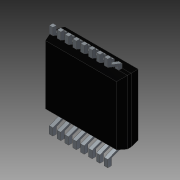
# Autodesk Inventor part: LTC6905
Saved by Autodesk Inventor 2013 (Build 170138000, 138)
## iProperties
Created: 2015-07-03
Part Number: LTC6905
Material: Ogólny
Document SubType Name: Modeling
Designer: terg
Density: 1 g/cm^3
Author: terg
Autodesk Inventor part; units mm, degrees
ref_plane "YZ Plane" through (0, 0, 0) normal (1, 0, 0) x (0, 1, 0)
ref_plane "XZ Plane" through (0, 0, 0) normal (0, 1, 0) x (-1, 0, 0)
sketch "Szkic1" plane through (0, 0, 0) normal (0, 1, 0) x (-1, 0, 0)
  line L0 (0, 0) -> (6.3, 0)
  line L1 (6.3, 0) -> (6.3, 5.3)
  line L2 (6.3, 5.3) -> (0, 5.3)
  line L3 (0, 5.3) -> (0, 0)
  dimension "d0" = 6.3
  dimension "d1" = 5.3
  constraints: 8 end point, 2 parallel, 1 horizontal, 1 perpendicular
  measures "d0" distance of L2.end L1.end
  measures "d1" distance of L1.end L0.end
extrude "Wyciągnięcie proste1" add sketch "Szkic1" along normal blind 1.7
chamfer "Faza1" distance 0.1 distance2 0.7 1 edges at (-3.15, 1.7, 0) measured on face at (-3.15, 1.7, 0.5)
chamfer "Faza2" distance 0.1 distance2 0.7 1 edges at (-3.15, 1.7, 5.3) measured on face at (-3.15, 1.7, 4.8)
chamfer "Faza3" distance 0.1 distance2 0.7 1 edges at (-6.3, 1.7, 2.65) measured on face at (-5.8, 1.7, 2.65)
chamfer "Faza4" distance 0.1 distance2 0.7 1 edges at (0, 1.7, 2.65) measured on face at (-0.5, 1.7, 2.65)
chamfer "Faza5" distance 0.7 distance2 0.2 1 edges at (-3.15, 0, 5.3) measured on face at (-3.15, 0.5, 5.3)
chamfer "Faza6" distance 0.7 distance2 0.2 1 edges at (-6.3, 0, 2.55) measured on face at (-6.3, 0.5, 2.55)
chamfer "Faza7" distance 0.7 distance2 0.2 1 edges at (-3.05, 0, 0) measured on face at (-3.05, 0.5, 0)
chamfer "Faza8" distance 0.7 distance2 0.2 1 edges at (0, 0, 2.65) measured on face at (0, 0.5, 2.65)
ref_plane "Płaszczyzna konstrukcyjna5" through (-3.15, 1, 0) normal (-1, 0, 0) x (0, 0, 1)
ref_plane "Płaszczyzna konstrukcyjna4" through (-3.475, 1, 0) normal (-1, 0, 0) x (0, 0, 1)
ref_plane "Płaszczyzna konstrukcyjna6" through (-3.8, 1, 0) normal (-1, 0, 0) x (0, 0, 1)
sketch "Szkic2" plane through (-3.475, 1, 0) normal (-1, 0, 0) x (0, 0, 1)
  line L0 (5.15, 0) -> (5.65, 0)
  line L1 (5.65, 0) -> (5.65, -0.3)
  line L2 (5.65, -0.3) -> (5.15, -0.3)
  line L3 (5.15, -0.3) -> (5.15, 0)
  line L4 (6, -0.9) -> (6.55, -0.9)
  line L5 (6.55, -0.9) -> (6.55, -1.2)
  line L6 (6.55, -1.2) -> (5.95, -1.2)
  line L7 (5.95, -1.2) -> (5.95, -1)
  line L8 (5.6, -0.3) -> (5.95, -1.2)
  line L9 (5.65, 0) -> (6, -0.9)
  line L10 (2.65, 0.4277) -> (2.65, -1.2185) construction
  line L11 (0.15, 0) -> (-0.35, 0)
  line L12 (-0.35, -0.3) -> (0.15, -0.3)
  line L13 (0.15, -0.3) -> (0.15, 0)
  line L14 (-0.7, -0.9) -> (-1.25, -0.9)
  line L15 (-1.25, -0.9) -> (-1.25, -1.2)
  line L16 (-1.25, -1.2) -> (-0.65, -1.2)
  line L17 (-0.3, -0.3) -> (-0.65, -1.2)
  line L18 (-0.35, 0) -> (-0.7, -0.9)
  line L19 (5.3, -0.3) -> (5.3, 0) projected
  line L20 (0, -0.3) -> (0, 0) projected
  point P0 (2.65, -0.55)
  dimension "d30" = 0.5
  dimension "d31" = 0.3
  dimension "d38" = 0.6
  dimension "d39" = 0.3
  dimension "d41" = 0.3
  dimension "d42" = 0.05
  dimension "d43" = 0.05
  dimension "d54" = 2.5
  dimension "d55" = 2.5
  dimension "d56" = 0
  dimension "d60" = 0
  dimension "d61" = 2.65
  dimension "d62" = 2.65
  dimension "d63" = 0.6
  constraints: 38 end point, 9 symmetric about line, 4 parallel, 2 horizontal, 2 perpendicular, 2 point on line
  measures "d30" distance of L1.end L2.end
  measures "d31" distance of L0.end L1.end
  measures "d38" distance of L5.end L6.end
  measures "d39" distance of L4.end L5.end
  measures "d41" distance between parallel lines of L7 L1
  measures "d42" distance from line of L1 L8.start
  measures "d43" distance from line of L4.start L7
  measures "d54" distance from line of L13.start L10
  measures "d55" distance between parallel lines of L10 L3
  measures "d56" distance from line of point (2.65, -0.55) L10
  measures "d60" distance from line of L19.end L0
  measures "d61" distance between parallel lines of L20 L10
  measures "d62" distance from line of L19 point (2.65, -0.55)
  measures "d63" distance between parallel lines of L2 L4
extrude "Wyciągnięcie proste3" add sketch "Szkic2" along normal mid plane 0.3
pattern_linear "Szyk prostokątny2" count 8 spacing 0.65 along (1, 0, 0) of "Wyciągnięcie proste3" first direction both ways yes
sketch "Szkic3" plane through (0, 1.7, 0) normal (0, 1, 0) x (1, 0, 0)
  line L0 (-6.2, -5.2) -> (-6.2, -0.1) projected
  line L1 (-0.1, -5.2) -> (-6.2, -5.2) projected
  point P0 (0, 0)
  point P1 (-5.7, -4.7)
  dimension "d70" = 0.5
  dimension "d71" = 0.5
  measures "d70" distance from line of L0 point (-5.7, -4.7)
  measures "d71" distance from line of L1 point (-5.7, -4.7)
hole "Otwór1" at (-5.7, 1.7, 4.7) direction (0, -1, 0) diameter 0.4 depth 0.1
equation "\"d43\" = d42"
equation "\"d61\" = d62"
